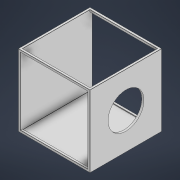
# Autodesk Inventor part: Body_prototype2
Saved by Autodesk Inventor 2021 (Build 250183000, 183)
## iProperties
Created: 2022-02-15
Part Number: Body_prototype2
Material: Generic
Document SubType Name: Modeling
Designer: utkaa
Density: 1 g/cm^3
Appearance: Default
Author: utkaa
Autodesk Inventor part; units mm, degrees
ref_plane "YZ Plane" through (0, 0, 0) normal (1, 0, 0) x (0, 1, 0)
ref_plane "XZ Plane" through (0, 0, 0) normal (0, 1, 0) x (-1, 0, 0)
ref_plane "XY Plane" through (0, 0, 0) normal (0, 0, 1) x (1, 0, 0)
sketch "Sketch2" plane through (0, 0, 0) normal (0, 1, 0) x (-1, 0, 0)
  line L0 (0, 0) -> (-1000, 0)
  line L1 (-1000, 0) -> (-1000, -1000)
  line L2 (-1000, -1000) -> (0, -1000)
  line L3 (0, -1000) -> (0, 0)
  dimension "d0" = 1000
  dimension "d1" = 1000
  constraints: 8 end point, 2 parallel, 1 horizontal, 1 perpendicular
  measures "d0" distance of L2.end L1.end
  measures "d1" distance of L0.end L1.end
extrude "Extrusion1" add sketch "Sketch2" along normal blind 1000
shell "Shell1" thickness 30 removed faces 0
sketch "Sketch3" plane through (0, 1000, 0) normal (0, 1, 0) x (1, 0, 0)
  line L0 (30, 30) -> (970, 30) projected
  line L1 (970, 30) -> (970, 970) projected
  line L2 (30, 30) -> (970, 30)
  line L3 (970, 30) -> (970, 970)
  line L4 (970, 970) -> (30, 970)
  line L5 (30, 970) -> (30, 30)
  point P0 (0, 0)
  constraints: 8 end point, 2 parallel, 1 horizontal, 1 perpendicular
extrude "Extrusion2" cut sketch "Sketch3" against normal blind 980
sketch "Sketch4" plane through (1000, 0, -1000) normal (0, 0, -1) x (-1, 0, 0)
  line L0 (30, 20) -> (30, 1000) projected
  line L1 (30, 30) -> (970, 30)
  line L2 (970, 30) -> (970, 970)
  line L3 (970, 970) -> (30, 970)
  line L4 (30, 970) -> (30, 30)
  line L5 (0, 0) -> (0, 1000) projected
  line L6 (0, 1000) -> (1000, 1000) projected
  point P0 (1000, 0)
  point P1 (30, 970)
  dimension "d7" = 940
  dimension "d8" = 940
  dimension "d9" = 30
  dimension "d10" = 30
  constraints: 8 end point, 2 parallel, 1 horizontal, 1 perpendicular, 1 point on line
  measures "d7" distance of L3.end L2.end
  measures "d8" distance of L1.end L2.end
  measures "d9" distance between parallel lines of L5 L0
  measures "d10" distance between parallel lines of L6 L3
extrude "Extrusion3" cut sketch "Sketch4" against normal blind 1000
fillet "Fillet1" radius 2 28 edges at (500, 1000, -1000) (500, 1000, 0) (500, 0, -1000) (500, 0, 0) (0, 500, 0) (0, 1000, -500) (0, 500, -1000) (500, 1000, -30) (30, 1000, -500) (500, 1000, -970) (500, 970, -970) (500, 30, -1000) (500, 30, -970) (500, 30, -30) (500, 30, 0) (500, 970, 0) (30, 500, 0) (30, 500, -1000) (0, 0, -500) (1000, 0, -500) (970, 500, 0) (1000, 500, 0) (970, 500, -1000) (1000, 500, -1000) (970, 1000, -500) (1000, 1000, -500) (500, 970, -1000) (30, 20, -500)
sketch "Sketch5" plane through (1000, 2, -2) normal (1, 0, 0) x (0, 0, -1)
  circle A0 centre (500, 500) radius 250
  line L0 (996, 0) -> (0, 0) projected
  line L1 (0, 0) -> (0, 996) projected
  point P0 (-2, -2)
  dimension "d14" = 500
  dimension "d15" = 500
  dimension "d16" = 500
  constraints: 1 centre point
  measures "d14" diameter of A0
  measures "d15" distance from line of A0.centre L0
  measures "d16" distance from line of L1 A0.centre
extrude "Extrusion4" cut sketch "Sketch5" against normal blind 100
body "Solid1"
